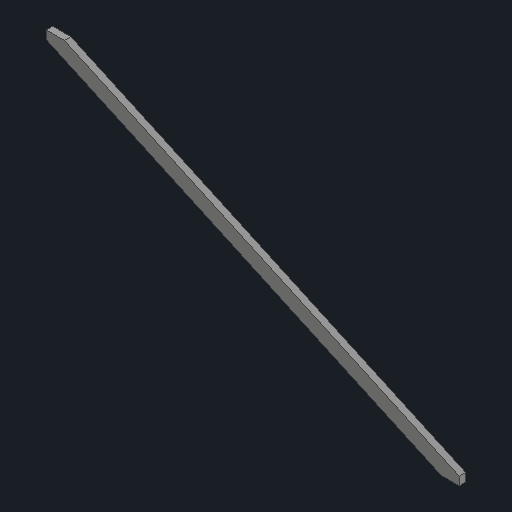
# Autodesk Inventor part: S_2x4x48b
Saved by Autodesk Inventor 2026 (Build 300175000, 175)
## iProperties
Created: 2024-09-16
Part Number: S_2x4x48b
Material: Generic
Document SubType Name: Modeling
Designer: User
Density: 1 g/cm^3
Appearance: Default
Author: User
Autodesk Inventor part; units mm, degrees
ref_plane "YZ Plane" through (0, 0, 0) normal (1, 0, 0) x (0, 1, 0)
ref_plane "XZ Plane" through (0, 0, 0) normal (0, 1, 0) x (-1, 0, 0)
ref_plane "XY Plane" through (0, 0, 0) normal (0, 0, 1) x (1, 0, 0)
sketch "Sketch1" plane through (0, 0, 0) normal (0, 0, 1) x (1, 0, 0)
  line L0 (0, 38.1) -> (-2438.4, 38.1) projected
  line L1 (0, 1149.35) -> (0, -1111.25) projected
  line L2 (0, 0) -> (-2438.4, 0) projected
  line L3 (-2438.4, 1149.35) -> (-2438.4, -1111.25) projected
  line L4 (0, 1149.35) -> (-2438.4, 1149.35) projected
  line L5 (0, 86.9483) -> (-2331.2129, 1149.35)
  line L6 (-2438.4, 1100.5017) -> (-107.1871, 38.1)
  line L7 (-2331.2129, 1149.35) -> (-2438.4, 1149.35)
  line L8 (-2438.4, 1100.5017) -> (-2438.4, 1149.35)
  line L9 (0, 86.9483) -> (0, 38.1)
  line L10 (-107.1871, 38.1) -> (0, 38.1)
  constraints: 12 end point, 4 point on line, 3 collinear, 1 parallel, 1 perpendicular, 1 other
extrude "Extrusion1" add sketch "Sketch1" against normal blind 38.1 contours L0 L6 L3 L4 L5 L1
body "Solid1"
